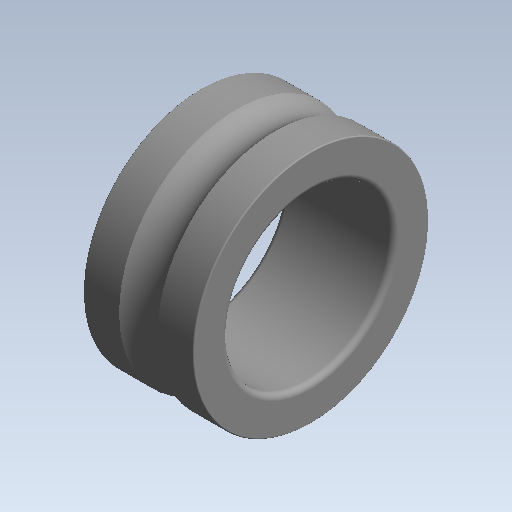
# Autodesk Inventor part: W 618/3_PART1
Saved by Autodesk Inventor 2021 (Build 250183000, 183)
## iProperties
Part Number: W 618/3_PART1
Material: Allgemein
Catalog Web Link: www.cadenas.de
Description: -Deep groove ball bearings
Vendor: SKF
Document SubType Name: Modeling
Designer: partserver
Manufacturer: SKF
Mass: 0.0137191 g
Surface Area: 0.598841 cm^2
Volume: 0.0137191 cm^3
Density: 1 g/cm^3
Appearance: PSOLRGB-175-175-175
Category: PARTsolutions
Company: SKF
PSOL_IDENT_0: {$CADENAS_DATA\23d-libs\skf\bearings_units_and_housings\ball_bearings\deep_groove_ball_bearings\bb1_
PSOL_IDENT_1: 001_101.prj},193 {VTYP=3D},{NB=W 618/3_PART1},{LINA=W 618/3_PART1},{NN=BB1_001_101_PART1},{NOPRJ=TRU
PSOL_IDENT_2: E},{DATE=19.12.2019 14:34:47},{GEOMDATE=18.12.2019 13:53:11},{VERSION=},{LINEID=16660},{WBVAR=},{WBN
PSOL_IDENT_3: UMERIC=}  {NB=W 618/3_PART1},{LINA=W 618/3_PART1},{KT=DUMMY},{PRODUCTID=},{DESIGNATION=W 618/3},{DD=
PSOL_IDENT_4: 3.000},{D=7.000},{B=2.000},{C=0.000},{DD1=4.28},{DD2=0.00},{D1=5.75},{D2=0.00},{D3=0.000},{D4=0.000}
PSOL_IDENT_5: ,{HH=MIN},{BB=0.000},{FF=0.00},{R0MAX=MIN},{R0=MIN},{R12=0.10},{PITCH=5.00},{DW=1.000},{DDAMIN=3.800
PSOL_IDENT_6: },{DDAMAX=MIN},{DDBMIN=MIN},{DDBMAX=MIN},{DBMIN=MIN},{DAMAX=6.200},{BBAMIN=MIN},{CAMAX=MIN},{RAMAX=0
PSOL_IDENT_7: .100},{LOAD1=0.178},{LOAD2=0.057},{LOAD3=0.002},{SPEED1=160000},{SPEED2=100000},{KR=0.020},{F0=7.100
PSOL_IDENT_8: },{Z=8},{II=1},{MASS=0.000},{BEARING=W 618/3},{RING=},{HELP=0.625},{HELP2=0.625},{DD1ALG=2.140},{YAL
PSOL_IDENT_9: G=2.140},{PITCH1=5.000},{DW1=1.000},{YALG1=2.875},{HALG1=0.625},{SH=2.140},{CU=0.200},{DESIGN=dgbbw}
PSOL_IDENT_10: ,{HALG=0.64},{B1=0},{SHIELDHELP=1}
NB: W 618/3_PART1
NT: Deep groove ball bearings
NBSYN: $DESIGNATION._PART1
LINA: W 618/3_PART1
CATALOG: SKF
SUPPLIER: SKF
ARTICLENO: W 618/3_PART1
BOMINFO: W 618/3_PART1
CREATOR: CADENAS GmbH
Title: W 618/3_PART1
Author: Cadenas PARTsolutions
Comments: Deep groove ball bearings
Autodesk Inventor part; units mm, degrees
ref_plane "YZ Plane" through (0, 0, 0) normal (1, 0, 0) x (0, 1, 0)
ref_plane "XZ Plane" through (0, 0, 0) normal (0, 1, 0) x (-1, 0, 0)
ref_plane "XY Plane" through (0, 0, 0) normal (0, 0, 1) x (1, 0, 0)
sketch "Sketch_10" plane through (0, 0, 0) normal (0, 0, 1) x (1, 0, 0)
  line L0 (50, 0) -> (-50, 0)
  line L1 (0, 2.12) -> (0, 1.6)
  arc A0 (0, 1.6) -> (0.1, 1.5) centre (0.1, 1.6) ccw
  line L2 (0.1, 1.5) -> (1.9, 1.5)
  arc A1 (1.9, 1.5) -> (2, 1.6) centre (1.9, 1.6) ccw
  line L3 (2, 1.6) -> (2, 2.12)
  arc A2 (2, 2.12) -> (1.98, 2.14) centre (1.98, 2.12) ccw
  line L4 (1.98, 2.14) -> (1.347, 2.14)
  arc A3 (0.653, 2.14) -> (1.347, 2.14) centre (1, 2.5) ccw
  line L5 (0.653, 2.14) -> (0.02, 2.14)
  arc A4 (0.02, 2.14) -> (0, 2.12) centre (0.02, 2.12) ccw
  constraints: 12 end point, 10 point on circle, 5 centre point
revolve "Revolution1" add sketch "Sketch_10" angle 360 about axis through (50, 0, 0) along (1, 0, 0)
body "Solid1"
